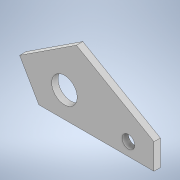
# Autodesk Inventor part: Assignment 1.5 - Slider Block
Saved by Autodesk Inventor 2021.1 (Build 251245000, 245)
## iProperties
Created: 2021-05-13
Part Number: Assignment 1.5 - Slider Block
Material: Generic
Document SubType Name: Modeling
Designer: as000166
Density: 1 g/cm^3
Appearance: Default
Author: as000166
Autodesk Inventor part; units mm, degrees
ref_plane "YZ Plane" through (0, 0, 0) normal (1, 0, 0) x (0, 1, 0)
ref_plane "XZ Plane" through (0, 0, 0) normal (0, 1, 0) x (-1, 0, 0)
ref_plane "XY Plane" through (0, 0, 0) normal (0, 0, 1) x (1, 0, 0)
sketch "Sketch1" plane through (0, 0, 0) normal (0, 0, 1) x (1, 0, 0)
  line L0 (114.3, 0) -> (114.3, 25.4)
  line L1 (114.3, 25.4) -> (37.3103, 69.85)
  line L2 (0, 0) -> (-19.05, 32.9956)
  line L3 (-19.05, 32.9956) -> (37.3103, 69.85)
  circle A0 centre (25.4, 25.4) radius 12.7
  circle A1 centre (88.9, 12.7) radius 6.35
  line L4 (0, 0) -> (114.3, 0)
  dimension "d1" = 25.4
  dimension "d2" = 88.9
  dimension "d4" = 38.1
  dimension "d8" = 25.4
  dimension "d11" = 12.7
  constraints: 10 end point, 2 centre point, 1 horizontal
  measures "d1" distance of L0.start L0.end
  measures "d2" distance of L0.end L1.end
  measures "d4" distance of L2.start L2.end
  measures "d8" diameter of A0
  measures "d11" diameter of A1
extrude "Extrusion1" add sketch "Sketch1" along normal blind 6.35
body "Solid1"
